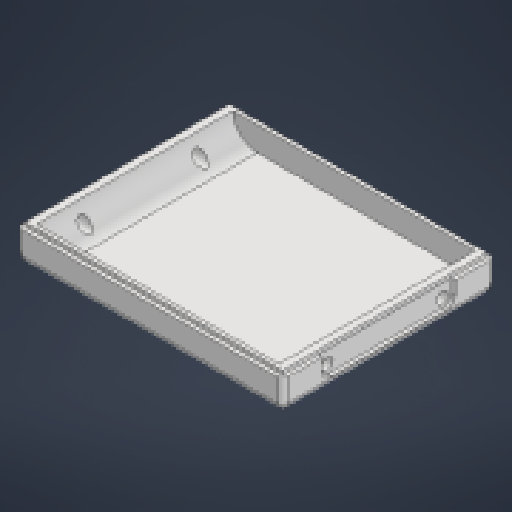
# Autodesk Inventor part: buttom case
Saved by Autodesk Inventor 2026.2 (Build 302298010, 298A)
## iProperties
Created: 2026-03-29
Part Number: buttom case
Material: 一般
Document SubType Name: Modeling
Designer: gavin
Density: 1 g/cm^3
Appearance: 預設
Author: gavin
## iProperties of the stored document buttom case_3D 列印.ipt
Created: 2026-03-29
Part Number: buttom case_3D 列印
Material: 一般
Document SubType Name: Modeling
Designer: gavin
Density: 1 g/cm^3
Appearance: 預設
Author: gavin
Autodesk Inventor part; units mm, degrees
ref_plane "YZ Plane" through (0, 0, 0) normal (1, 0, 0) x (0, 1, 0)
ref_plane "XZ Plane" through (0, 0, 0) normal (0, 1, 0) x (-1, 0, 0)
ref_plane "XY Plane" through (0, 0, 0) normal (0, 0, 1) x (1, 0, 0)
sketch "草圖1" plane through (0, 0, 0) normal (0, 1, 0) x (-1, 0, 0)
  line L0 (25, 40) -> (-25, 40)
  line L1 (-25, 40) -> (-25, -40)
  line L2 (-25, -40) -> (25, -40)
  line L3 (25, -40) -> (25, 40)
  line L4 (25, 40) -> (-25, -40) construction
  line L5 (-25, 40) -> (25, -40) construction
  point P0 (0, 0)
  dimension "d0" = 50
  dimension "d1" = 80
  constraints: 12 end point, 2 midpoint, 2 parallel, 1 horizontal, 1 perpendicular
  measures "d0" distance of L2.end L1.end
  measures "d1" distance of L1.end L0.end
extrude "擠出1" add sketch "草圖1" along normal blind 3
sketch "草圖2" plane through (0, 3, 0) normal (0, 1, 0) x (1, 0, 0)
  line L0 (25, -40) -> (25, 40) projected
  line L1 (25, 40) -> (-25, 40) projected
  line L2 (-25, 40) -> (-25, -40) projected
  line L3 (-25, -40) -> (25, -40) projected
  line L4 (-22, -37) -> (-22, 37)
  line L5 (-22, 37) -> (22, 37)
  line L6 (22, 37) -> (22, -37)
  line L7 (22, -37) -> (-22, -37)
  point P0 (0, 0)
  dimension "d4" = 3
  constraints: 8 end point, 3 other
  measures "d4" distance between parallel lines of L2 L4
extrude "擠出2" add sketch "草圖2" along normal blind 9.125
sketch "草圖3" plane through (-22, 3, -37) normal (0, 0, 1) x (1, 0, 0)
  line L0 (44, 0) -> (0, 0) projected
  line L1 (44, 0) -> (44, 9.125) projected
  line L2 (0, 9.125) -> (44, 9.125) projected
  line L3 (0, 0) -> (0, 9.125) projected
  circle A0 centre (-41.875, 9.125) radius 9.125
  circle A1 centre (-23.625, 9.125) radius 9.125
  circle A2 centre (-5.375, 9.125) radius 9.125
  circle A3 centre (12.875, 9.125) radius 9.125
  circle A4 centre (31.125, 9.125) radius 9.125
  point P0 (22, -3)
  point P1 (40.25, 9.125)
  point P2 (31.125, 0)
  point P3 (10.5, 0)
  point P4 (1.375, 9.125)
  point P5 (12.875, 0)
  point P6 (3.75, 9.125)
  dimension "d7" = 18.25
  dimension "d11" = 18.25
  dimension "d16" = 12.875
  constraints: 5 centre point, 1 horizontal, 1 point on line, 8 other
  measures "d7" diameter of A0
  measures "d11" distance of A0.centre A1.centre
  measures "d16" distance from line of A4.centre L1
extrude "擠出3" add sketch "草圖3" along normal through all contours L0 A4 L2 L1 | L0 L3 A2 A3 | A2 L3 L2 picked at (0.5235, 4.6943)
sketch "草圖4" plane through (0, 12.125, 0) normal (0, 1, 0) x (1, 0, 0)
  line L0 (-25, -40) -> (25, -40) projected
  line L1 (25, -40) -> (25, 40) projected
  line L2 (25, 40) -> (-25, 40) projected
  line L3 (-25, 40) -> (-25, -40) projected
  line L4 (23.5, -38.5) -> (-23.5, -38.5)
  line L5 (-23.5, -38.5) -> (-23.5, 38.5)
  line L6 (-23.5, 38.5) -> (23.5, 38.5)
  line L7 (23.5, 38.5) -> (23.5, -38.5)
  line L8 (-23.45, -38.45) -> (23.45, -38.45)
  line L9 (23.45, -38.45) -> (23.45, 38.45)
  line L10 (23.45, 38.45) -> (-23.45, 38.45)
  line L11 (-23.45, 38.45) -> (-23.45, -38.45)
  point P0 (0, 0)
  dimension "d19" = 1.5
  dimension "d20" = 0.05
  constraints: 16 end point, 6 other
  measures "d19" distance between parallel lines of L0 L4
  measures "d20" distance between parallel lines of L4 L8
extrude "擠出4" cut sketch "草圖4" against normal blind 1.51 contours L3 L2 L1 L0 | L4 L5 L6 L7
sketch "草圖5" plane through (25, 0, 40) normal (1, 0, 0) x (0, 0, -1)
  circle A0 centre (18.3, 5.925) radius 1.65 projected
  circle A1 centre (61.7, 5.925) radius 1.65 projected
  line L0 (28.79, 20.925) -> (15, 20.925) projected
  line L1 (15, 20.925) -> (15, 27.625) projected
  line L2 (15, 27.625) -> (28.79, 27.625) projected
  line L3 (28.79, 27.625) -> (28.79, 20.925) projected
  line L4 (51.21, 20.925) -> (51.21, 27.625) projected
  line L5 (51.21, 27.625) -> (65, 27.625) projected
  line L6 (65, 27.625) -> (65, 20.925) projected
  line L7 (65, 20.925) -> (51.21, 20.925) projected
  line L8 (15, 10.625) -> (2, 10.625) projected
  line L9 (15, 10.625) -> (15, 5.925) projected
  arc A2 (15, 5.925) -> (18.3, 2.625) centre (18.3, 5.925) ccw projected
  line L10 (18.3, 2.625) -> (61.7, 2.625) projected
  arc A3 (61.7, 2.625) -> (65, 5.925) centre (61.7, 5.925) ccw projected
  line L11 (65, 5.925) -> (65, 10.625) projected
  line L12 (78, 10.625) -> (65, 10.625) projected
  line L13 (15, 10.625) -> (65, 10.625)
  line L14 (80, 10.615) -> (0, 10.615) projected
  arc A4 (14.9, 5.925) -> (18.3, 2.525) centre (18.3, 5.925) ccw
  line L15 (14.9, 5.925) -> (14.9, 10.525)
  line L16 (14.9, 10.525) -> (-0.1, 10.525)
  line L17 (-0.1, 10.525) -> (-0.1, 30.725)
  line L18 (-0.1, 30.725) -> (80.1, 30.725)
  line L19 (80.1, 30.725) -> (80.1, 10.525)
  line L20 (80.1, 10.525) -> (65.1, 10.525)
  line L21 (65.1, 10.525) -> (65.1, 5.925)
  arc A5 (61.7, 2.525) -> (65.1, 5.925) centre (61.7, 5.925) ccw
  line L22 (61.7, 2.525) -> (18.3, 2.525)
  line L23 (14.9, 10.525) -> (14.9, 10.615)
  line L24 (65.1, 10.525) -> (65.1, 10.615)
  line L25 (78, 28.625) -> (78, 10.625) projected
  line L26 (2, 10.625) -> (2, 28.625) projected
  line L27 (46.97, 28.625) -> (46.97, 20.925) projected
  line L28 (46.97, 20.925) -> (33.03, 20.925) projected
  line L29 (33.03, 20.925) -> (33.03, 28.625) projected
  line L30 (46.97, 28.625) -> (78, 28.625) projected
  line L31 (2, 28.625) -> (33.03, 28.625) projected
  point P0 (40, 0)
  dimension "d23" = 0.1
  constraints: 22 end point, 4 point on circle, 2 centre point, 2 perpendicular, 2 point on line, 1 parallel, 5 other
  measures "d23" radial gap between concentric circles of A2 A4
extrude "擠出5" cut sketch "草圖5" against normal blind 1.51 contours A0 | A1 | L14 L11 A3 L10 A2 L9 | L9 A2 L10 A3 L11 L14 L24 L21 A5 L22 A4 L15 L23
mirror "鏡射1" about plane through (0, 0, 0) normal (1, 0, 0) of "擠出5"
sketch "草圖6" plane through (23.49, 0, 40) normal (1, 0, 0) x (0, 0, -1)
  circle A0 centre (18.3, 5.925) radius 1.65 projected
  circle A1 centre (61.7, 5.925) radius 1.65 projected
  circle A2 centre (18.3, 5.925) radius 2.165
  circle A3 centre (61.7, 5.925) radius 2.165
  point P0 (40, 0)
  dimension "d26" = 4.33
  dimension "d27" = 4.33
  constraints: 2 centre point, 2 coincident
  measures "d26" diameter of A2
  measures "d27" diameter of A3
extrude "擠出6" cut sketch "草圖6" against normal through all contours A0 | A1 | A2 | A3
fillet "圓角1" radius 2 7 edges at (-25, 5.3075, 40) (0, 0, 40) (25, 5.3075, 40) (25, 0, 0) (0, 0, -40) (-25, 0, 0) (-25, 5.3075, -40)
fillet "圓角2" radius 2 2 edges at (24.4142, 0.5858, -39.4142) (25, 6.3075, -40)
ref_plane "工作平面1" through (-22, 5.925, 25.1) normal (-1, 0, 0) x (0, 0, 1)
sketch "草圖7" plane through (-22, 5.925, 25.1) normal (-1, 0, 0) x (0, 0, 1)
  circle A0 centre (-46.8, 0) radius 2.165 projected
  circle A1 centre (-3.4, 0) radius 2.165 projected
  line L0 (-46.8, 3.4641) -> (-43.8, 1.7321)
  line L1 (-43.8, 1.7321) -> (-43.8, -1.7321)
  line L2 (-43.8, -1.7321) -> (-46.8, -3.4641)
  line L3 (-46.8, -3.4641) -> (-49.8, -1.7321)
  line L4 (-49.8, -1.7321) -> (-49.8, 1.7321)
  line L5 (-49.8, 1.7321) -> (-46.8, 3.4641)
  line L6 (-3.4, 3.4641) -> (-0.4, 1.7321)
  line L7 (-0.4, 1.7321) -> (-0.4, -1.7321)
  line L8 (-0.4, -1.7321) -> (-3.4, -3.4641)
  line L9 (-3.4, -3.4641) -> (-6.4, -1.7321)
  line L10 (-6.4, -1.7321) -> (-6.4, 1.7321)
  line L11 (-6.4, 1.7321) -> (-3.4, 3.4641)
  line L12 (-49.8, 1.7321) -> (-49.8, 7.8843)
  line L13 (-50.2, 4.69) -> (-50.2, 0) projected
  line L14 (-49.8, 7.8843) -> (-43.8, 7.8843)
  line L15 (-43.8, 7.8843) -> (-43.8, 1.7321)
  line L16 (-6.4, 1.7321) -> (-6.4, 7.8843)
  line L17 (-6.4, 7.8843) -> (-0.4, 7.8843)
  line L18 (-0.4, 7.8843) -> (-0.4, 1.7321)
  point P0 (-25.1, -5.925)
  dimension "d33" = 6
  dimension "d34" = 6
  constraints: 36 end point, 2 coincident, 2 parallel, 2 perpendicular, 2 point on line, 1 collinear, 26 other
  measures "d33" distance between parallel lines of L1 L4
  measures "d34" distance between parallel lines of L7 L10
extrude "擠出7" cut sketch "草圖7" against normal blind 2.5
ref_plane "工作平面2" through (0, 5.925, -25.1) normal (1, 0, 0) x (0, 0, -1)
mirror "鏡射2" about plane through (0, 5.925, -25.1) normal (1, 0, 0) of "擠出7"
